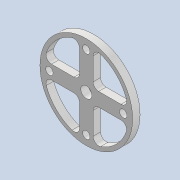
# Autodesk Inventor part: tp_wheel_1
Saved by Autodesk Inventor 2020 (Build 240168000, 168)
## iProperties
Created: 2021-10-11
Part Number: tp_wheel_1
Material: Generic
Document SubType Name: Modeling
Designer: Shuang Peng
Density: 1 g/cm^3
Appearance: Default
Author: Shuang Peng
Autodesk Inventor part; units mm, degrees
ref_plane "YZ Plane" through (0, 0, 0) normal (1, 0, 0) x (0, 1, 0)
ref_plane "XZ Plane" through (0, 0, 0) normal (0, 1, 0) x (-1, 0, 0)
ref_plane "XY Plane" through (0, 0, 0) normal (0, 0, 1) x (1, 0, 0)
sketch "Sketch1" plane through (0, 0, 0) normal (0, 0, 1) x (1, 0, 0)
  circle A0 centre (-10, 0) radius 1 projected
  circle A1 centre (0, 10) radius 1 projected
  circle A2 centre (0, -10) radius 1 projected
  circle A3 centre (10, 0) radius 1 projected
  circle A4 centre (0, 0) radius 1.5 projected
  arc A5 (10.8355, 3.8525) -> (3.8525, 10.8355) centre (0, 0) ccw projected
  arc A6 (9.4222, 1.85) -> (10.8355, 3.8525) centre (9.4222, 3.35) ccw projected
  line L0 (9.4222, 1.85) -> (3.35, 1.85) projected
  arc A7 (1.85, 3.35) -> (3.35, 1.85) centre (3.35, 3.35) ccw projected
  line L1 (1.85, 3.35) -> (1.85, 9.4222) projected
  arc A8 (3.8525, 10.8355) -> (1.85, 9.4222) centre (3.35, 9.4222) ccw projected
  line L2 (-1.85, 9.4222) -> (-1.85, 3.35) projected
  arc A9 (-3.35, 1.85) -> (-1.85, 3.35) centre (-3.35, 3.35) ccw projected
  line L3 (-3.35, 1.85) -> (-9.4222, 1.85) projected
  arc A10 (-10.8355, 3.8525) -> (-9.4222, 1.85) centre (-9.4222, 3.35) ccw projected
  arc A11 (-3.8525, 10.8355) -> (-10.8355, 3.8525) centre (0, 0) ccw projected
  arc A12 (-1.85, 9.4222) -> (-3.8525, 10.8355) centre (-3.35, 9.4222) ccw projected
  line L4 (3.35, -1.85) -> (9.4222, -1.85) projected
  arc A13 (10.8355, -3.8525) -> (9.4222, -1.85) centre (9.4222, -3.35) ccw projected
  arc A14 (3.8525, -10.8355) -> (10.8355, -3.8525) centre (0, 0) ccw projected
  arc A15 (1.85, -9.4222) -> (3.8525, -10.8355) centre (3.35, -9.4222) ccw projected
  line L5 (1.85, -9.4222) -> (1.85, -3.35) projected
  arc A16 (3.35, -1.85) -> (1.85, -3.35) centre (3.35, -3.35) ccw projected
  line L6 (-1.85, -3.35) -> (-1.85, -9.4222) projected
  arc A17 (-3.8525, -10.8355) -> (-1.85, -9.4222) centre (-3.35, -9.4222) ccw projected
  arc A18 (-10.8355, -3.8525) -> (-3.8525, -10.8355) centre (0, 0) ccw projected
  arc A19 (-9.4222, -1.85) -> (-10.8355, -3.8525) centre (-9.4222, -3.35) ccw projected
  line L7 (-9.4222, -1.85) -> (-3.35, -1.85) projected
  arc A20 (-1.85, -3.35) -> (-3.35, -1.85) centre (-3.35, -3.35) ccw projected
  circle A21 centre (0, 0) radius 12.55 projected
  point P0 (0, 0)
extrude "Extrusion1" add sketch "Sketch1" along normal blind 2
sketch "Sketch2" plane through (0, 0, 2) normal (0, 0, 1) x (1, 0, 0)
  circle A0 centre (0, 0) radius 1.5 projected
  circle A1 centre (0, 0) radius 4
  point P0 (0, 0)
  dimension "d2" = 8
  constraints: 1 centre point, 1 coincident
  measures "d2" diameter of A1
extrude "Extrusion2" add sketch "Sketch2" along normal blind 6
sketch "Sketch3" plane through (0, 0, 8) normal (0, 0, 1) x (1, 0, 0)
  line L0 (0, -4) -> (0, 4) construction
  line L1 (0.25, -4) -> (0.25, 4)
  line L2 (-0.25, 4) -> (-0.25, -4)
  arc A0 (-0.25, -4) -> (0.25, -4) centre (0, -4) ccw
  arc A1 (0.25, 4) -> (-0.25, 4) centre (0, 4) ccw
  point P0 (0, 0)
  dimension "d5" = 4
  dimension "d6" = 0.5
  constraints: 8 end point, 4 point on circle, 4 tangent, 2 centre point, 1 midpoint, 1 parallel, 1 vertical
  measures "d5" distance of point (0, 0) L0.end
  measures "d6" diameter of A1
extrude "Extrusion3" cut sketch "Sketch3" against normal blind 6
fillet "Fillet1" radius 0.5 12 edges at (3.4482, -1.85, 2) (1.85, -3.4482, 2) (2.2893, -2.2893, 2) (1.85, 3.4482, 2) (3.4482, 1.85, 2) (2.2893, 2.2893, 2) (-3.4482, 1.85, 2) (-1.85, 3.4482, 2) (-2.2893, 2.2893, 2) (-1.85, -3.4482, 2) (-3.4482, -1.85, 2) (-2.2893, -2.2893, 2)
body "Solid1"
